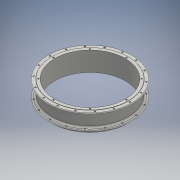
# Autodesk Inventor part: Pièce1
Saved by Autodesk Inventor 2016 (Build 200138000, 138)
## iProperties
Created: 2015-11-15
Part Number: Pièce1
Material: Générique
Document SubType Name: Modeling
Designer: Cyril
Density: 1 g/cm^3
Appearance: Par défaut
Author: Cyril
Autodesk Inventor part; units mm, degrees
ref_plane "YZ Plane" through (0, 0, 0) normal (1, 0, 0) x (0, 1, 0)
ref_plane "XZ Plane" through (0, 0, 0) normal (0, 1, 0) x (-1, 0, 0)
ref_plane "XY Plane" through (0, 0, 0) normal (0, 0, 1) x (1, 0, 0)
sketch "Esquisse1" plane through (0, 0, 0) normal (1, 0, 0) x (0, 1, 0)
  line L0 (0, 0) -> (111, 0) construction
  line L1 (111, 0) -> (111, 15.5)
  arc A0 (116, 20.5) -> (111, 15.5) centre (116, 15.5) ccw
  line L2 (116, 20.5) -> (120.5, 20.5)
  arc A1 (120.5, 20.5) -> (120.5, 23.5) centre (120.5, 22) ccw
  line L3 (111, 0) -> (111, -15.5)
  arc A2 (111, -15.5) -> (116, -20.5) centre (116, -15.5) ccw
  line L4 (116, -20.5) -> (120.5, -20.5)
  arc A3 (120.5, -23.5) -> (120.5, -20.5) centre (120.5, -22) ccw
  line L5 (120.5, 23.5) -> (111.5, 23.5)
  arc A4 (111, 24) -> (111.5, 23.5) centre (111.5, 24) ccw
  line L6 (111, 24) -> (102.5, 24)
  arc A5 (113, -23.5) -> (111, -25.5) centre (113, -25.5) ccw
  line L7 (113, -23.5) -> (120.5, -23.5)
  line L8 (111, -25.5) -> (111, -32.5)
  line L9 (111, -32.5) -> (102.5, -32.5)
  line L10 (102.5, 24) -> (102.5, -32.5)
  line L11 (0, 24) -> (0, -32.5) construction
  dimension "d0" = 1.5
  dimension "d1" = 5
  dimension "d2" = 2
  dimension "d3" = 0.5
  dimension "d27" = 120.5
  dimension "d28" = 111
  dimension "d29" = 47
  dimension "d30" = 102.5
  dimension "d31" = 56.5
  constraints: 24 end point, 12 point on circle, 7 tangent, 6 centre point, 6 horizontal, 6 point on line, 6 symmetric about line, 4 vertical, 2 other
  measures "d0" radius of A1
  measures "d1" radius of A0
  measures "d2" radius of A5
  measures "d3" radius of A4
  measures "d27" horizontal distance of L0.start A1.centre
  measures "d28" horizontal distance of L0.start L6.start
  measures "d29" distance between parallel lines of L7 L5
  measures "d30" distance between parallel lines of L11 L10
  measures "d31" distance between parallel lines of L9 L6
revolve "Révolution1" add sketch "Esquisse1" angle 360 about axis through (0, 0, 24) along (0, 0, -1)
sketch "Esquisse2" plane through (0, 0, 23.5) normal (0, 0, 1) x (1, 0, 0)
  circle A0 centre (-116, 0) radius 2.1
  circle A1 centre (-109.0043, -39.6743) radius 2.1
  circle A2 centre (-88.8612, -74.5634) radius 2.1
  circle A3 centre (-58, -100.4589) radius 2.1
  circle A4 centre (-20.1432, -114.2377) radius 2.1
  circle A5 centre (20.1432, -114.2377) radius 2.1
  circle A6 centre (58, -100.4589) radius 2.1
  circle A7 centre (88.8612, -74.5634) radius 2.1
  circle A8 centre (109.0043, -39.6743) radius 2.1
  circle A9 centre (116, 0) radius 2.1
  circle A10 centre (109.0043, 39.6743) radius 2.1
  circle A11 centre (88.8612, 74.5634) radius 2.1
  circle A12 centre (58, 100.4589) radius 2.1
  circle A13 centre (20.1432, 114.2377) radius 2.1
  circle A14 centre (-20.1432, 114.2377) radius 2.1
  circle A15 centre (-58, 100.4589) radius 2.1
  circle A16 centre (-88.8612, 74.5634) radius 2.1
  circle A17 centre (-109.0043, 39.6743) radius 2.1
  line L0 (-116, 0) -> (116, 0) construction
  point P0 (0, 0)
  dimension "d9" = 4.2
  dimension "d12" = 360
  dimension "d14" = 232
  constraints: 18 centre point, 2 end point, 1 horizontal, 37 other
  measures "d9" diameter of A0
  measures "d14" distance of L0.start L0.end
extrude "Extrusion1" cut sketch "Esquisse2" against normal blind 15
sketch "Esquisse3" plane through (0, 0, -23.5) normal (0, 0, -1) x (-1, 0, 0)
  circle A0 centre (0, 116) radius 2.1
  line L0 (0, 0) -> (0, 116) construction
  circle A1 centre (-39.6743, 109.0043) radius 2.1
  circle A2 centre (-74.5634, 88.8612) radius 2.1
  circle A3 centre (-100.4589, 58) radius 2.1
  circle A4 centre (-114.2377, 20.1432) radius 2.1
  circle A5 centre (-114.2377, -20.1432) radius 2.1
  circle A6 centre (-100.4589, -58) radius 2.1
  circle A7 centre (-74.5634, -88.8612) radius 2.1
  circle A8 centre (-39.6743, -109.0043) radius 2.1
  circle A9 centre (0, -116) radius 2.1
  circle A10 centre (39.6743, -109.0043) radius 2.1
  circle A11 centre (74.5634, -88.8612) radius 2.1
  circle A12 centre (100.4589, -58) radius 2.1
  circle A13 centre (114.2377, -20.1432) radius 2.1
  circle A14 centre (114.2377, 20.1432) radius 2.1
  circle A15 centre (100.4589, 58) radius 2.1
  circle A16 centre (74.5634, 88.8612) radius 2.1
  circle A17 centre (39.6743, 109.0043) radius 2.1
  dimension "d19" = 4.2
  dimension "d22" = 360
  dimension "d24" = 232
  constraints: 18 centre point, 2 end point, 1 vertical, 37 other
  measures "d19" diameter of A0
  measures "d24" distance of A9.centre L0.end
extrude "Extrusion2" cut sketch "Esquisse3" against normal blind 10
sketch "Esquisse4" plane through (0, 0, 24) normal (0, 0, 1) x (1, 0, 0)
  line L0 (0, -170.8) -> (0, 170.8) projected
  point P0 (0, 0)
  point P1 (0, 106)
  point P2 (-74.9533, 74.9533)
  point P3 (-106, 0)
  point P4 (-74.9533, -74.9533)
  point P5 (0, -106)
  point P6 (74.9533, -74.9533)
  point P7 (106, 0)
  point P8 (74.9533, 74.9533)
  dimension "d34" = 360
  dimension "d36" = 212
  constraints: 1 point on line, 9 other
  measures "d36" distance of point (0, -106) point (0, 106)
hole "Perçage1" at (0, 106, 24) at (-74.9533, 74.9533, 24) at (-106, 0, 24) at (-74.9533, -74.9533, 24) at (0, -106, 24) at (74.9533, -74.9533, 24) at (106, 0, 24) at (74.9533, 74.9533, 24) direction (0, 0, -1) diameter 4.134 depth 14 tip angle 118 thread size "M5x0.8" class "6H" standard "ISO Metric profile"
sketch "Esquisse5" plane through (0, 0, -32.5) normal (0, 0, -1) x (-1, 0, 0)
  line L0 (0, 0) -> (0, 106) construction
  point P0 (-74.9533, 74.9533)
  point P1 (-106, 0)
  point P2 (-74.9533, -74.9533)
  point P3 (0, -106)
  point P4 (74.9533, -74.9533)
  point P5 (106, 0)
  point P6 (74.9533, 74.9533)
  dimension "d46" = 360
  dimension "d48" = 212
  constraints: 2 end point, 1 vertical, 9 other
  measures "d48" distance of point (0, -106) L0.end
hole "Perçage2" at (0, 106, -32.5) at (74.9533, 74.9533, -32.5) at (106, 0, -32.5) at (74.9533, -74.9533, -32.5) at (0, -106, -32.5) at (-74.9533, -74.9533, -32.5) at (-106, 0, -32.5) at (-74.9533, 74.9533, -32.5) direction (0, 0, 1) diameter 4.134 depth 14 tip angle 118 thread size "M5x0.8" class "6H" standard "ISO Metric profile"
